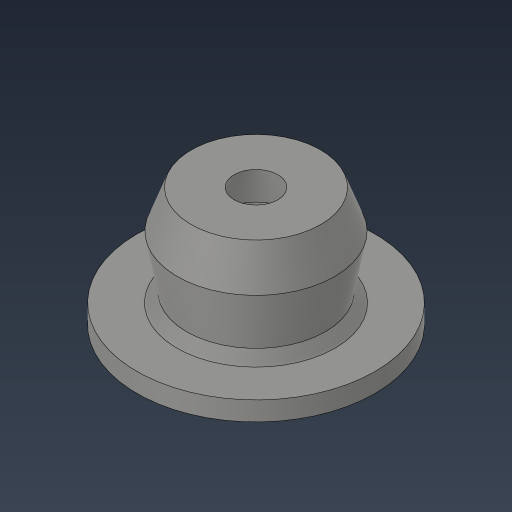
# Autodesk Inventor part: Druckknopf
Saved by Autodesk Inventor 2023.1 (Build 271208000, 208)
## iProperties
Part Number: Druckknopf
Material: Gummi, Silikon
Document SubType Name: Modeling
Designer: rYan
Density: 1.25 g/cm^3
Appearance: Glatt - Mittelgrau
Mass: 0.208264 g
Surface Area: 2.92575 cm^2
Volume: 0.166611 cm^3
Author: rYan
Autodesk Inventor part; units mm, degrees
ref_plane "YZ Plane" through (0, 0, 0) normal (1, 0, 0) x (0, 1, 0)
ref_plane "XZ Plane" through (0, 0, 0) normal (0, 1, 0) x (-1, 0, 0)
ref_plane "XY Plane" through (0, 0, 0) normal (0, 0, 1) x (1, 0, 0)
sketch "Skizze1" plane through (0, 0, 0) normal (0, 1, 0) x (-1, 0, 0)
  line L0 (-6, 0) -> (1, 0) construction
  line L1 (-1.0415, 0) -> (-1.5, 2.6)
  line L2 (-1.5, 2.6) -> (-0.9176, 4.2)
  line L3 (-0.9176, 4.2) -> (-2.7176, 4.2)
  line L4 (-2.7176, 4.2) -> (-3.3, 2.6)
  line L5 (-3.3, 2.6) -> (-2.9121, 0.4)
  line L6 (-1.5, 2.6) -> (-3.3, 2.6) construction
  line L7 (-2.9121, 0.4) -> (-3.3121, 0)
  line L8 (-3.3121, 0) -> (-5, 0)
  line L9 (-5, 0) -> (-5, -0.8)
  line L10 (-5, -0.8) -> (0, -0.8)
  line L11 (0, -0.8) -> (0, 0)
  line L12 (-1.0415, 0) -> (0, 0)
  line L13 (0, -0.8) -> (0, 4.2)
  dimension "d0" = 80
  dimension "d1" = 70
  dimension "d2" = 1.8
  dimension "d3" = 2.6
  dimension "d4" = 1.6
  dimension "d21" = 45
  dimension "d22" = 0.4
  dimension "d23" = 0.8
  dimension "d24" = 10
  dimension "d26" = 6.6
  constraints: 26 end point, 4 point on line, 2 horizontal, 2 parallel, 2 perpendicular, 2 vertical, 1 collinear
  measures "d0" angle of L5 L0
  measures "d1" angle of L4 L6
  measures "d2" distance of L1.end L4.end
  measures "d3" distance between parallel lines of L0 L6
  measures "d4" distance between parallel lines of L6 L3
  measures "d21" angle of L0 L7
  measures "d22" distance from line of L0 L5.end
  measures "d23" distance of L8.end L9.end
  measures "d24" diameter of L9 L13
  measures "d26" diameter of L4.end L13
revolve "Umdrehung1" add sketch "Skizze1" angle 360 about axis through (0, 0, -0.8) along (0, 0, 1)
